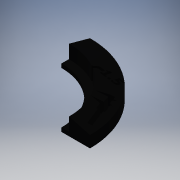
# Autodesk Inventor part: Mentor-CAD ring
Saved by Autodesk Inventor 2016 (Build 200138000, 138)
## iProperties
Created: 2016-02-20
Part Number: Mentor-CAD ring
Material: Generic
Document SubType Name: Modeling
Designer: RoksBot
Density: 1 g/cm^3
Appearance: Fine Textured - Black
Author: RoksBot
Autodesk Inventor part; units mm, degrees
ref_plane "YZ Plane" through (0, 0, 0) normal (1, 0, 0) x (0, 1, 0)
ref_plane "XZ Plane" through (0, 0, 0) normal (0, 1, 0) x (-1, 0, 0)
ref_plane "XY Plane" through (0, 0, 0) normal (0, 0, 1) x (1, 0, 0)
sketch "Sketch1" plane through (0, 0, 0) normal (0, 0, 1) x (1, 0, 0)
  line L0 (0, 0) -> (0, 8.6646) construction
  line L1 (20.9931, 1.27) -> (20.9931, 5.715)
  line L2 (20.9931, 5.715) -> (27.9781, 3.81)
  line L3 (27.9781, 3.81) -> (27.9781, 0)
  line L4 (27.9781, 0) -> (20.9931, 0)
  line L5 (20.9931, 1.27) -> (18.4531, 1.27)
  line L6 (18.4531, 1.27) -> (18.4531, 0)
  line L7 (18.4531, 0) -> (20.9931, 0)
  dimension "d0" = 20.9931
  dimension "d1" = 4.445
  dimension "d2" = 1.27
  dimension "d3" = 2.54
  dimension "d4" = 3.81
  dimension "d5" = 6.985
  constraints: 16 end point, 2 parallel, 2 perpendicular, 2 vertical, 1 horizontal, 1 horizontal alignment
  measures "d0" distance between parallel lines of L0 L1
  measures "d1" distance from line of L5 L1.end
  measures "d2" distance of L5.end L6.end
  measures "d3" distance between parallel lines of L1 L6
  measures "d4" distance of L2.end L3.end
  measures "d5" distance between parallel lines of L1 L3
revolve "Revolution1" add sketch "Sketch1" angle 360 about axis through (0, 0, 0) along (0, 1, 0)
sketch "Sketch2" plane through (0, 1.27, 0) normal (0, 1, 0) x (1, 0, 0)
  circle A0 centre (0, 0) radius 20.9931 projected
  circle A1 centre (0, 0) radius 27.9781 projected
  circle A2 centre (0, 0) radius 18.4531 projected
  line L0 (-4.2505, -7.1349) -> (4.1315, -7.1349) projected
  circle A3 centre (0, 0) radius 19.685 projected
  line L1 (-12.7595, -2.2222) -> (-12.7595, -29.7716) construction
  line L2 (12.6405, -2.2222) -> (12.6405, -30.8961) construction
  line L3 (-12.7549, -7.1349) -> (-31.6502, -7.1349) construction
  line L4 (0, 0) -> (17.3317, 30.0193) construction
  line L5 (-18.5741, 9.7833) -> (-25.4, 9.7833)
  line L6 (-18.8949, 9.1483) -> (-25.4, 9.1483)
  line L7 (-25.4, 9.1483) -> (-25.4, 9.7833)
  line L8 (-19.8553, -6.8174) -> (-25.4, -6.8174)
  line L9 (-25.4, -6.8174) -> (-25.4, -7.4524)
  line L10 (-25.4, -7.4524) -> (-19.6258, -7.4524)
  line L11 (0.1351, 9.4658) -> (-31.517, 9.4658) construction
  line L12 (-24.13, 9.1483) -> (-22.86, 6.9486)
  line L13 (-22.86, 6.9486) -> (-25.4, 6.9486)
  line L14 (-25.4, 6.9486) -> (-24.13, 9.1483)
  line L15 (-24.13, -6.8174) -> (-25.4, -4.6177)
  line L16 (-25.4, -4.6177) -> (-22.86, -4.6177)
  line L17 (-22.86, -4.6177) -> (-24.13, -6.8174)
  line L18 (-29.0818, 1.1654) -> (-16.5563, 1.1654) construction
  line L19 (-24.13, 7.6818) -> (-24.13, -5.3509) construction
  line L20 (-23.8125, 2.4354) -> (-24.4475, 2.4354)
  line L21 (-24.4475, 2.4354) -> (-24.4475, 6.9486)
  line L22 (-24.4475, 6.9486) -> (-23.8125, 6.9486)
  line L23 (-23.8125, 6.9486) -> (-23.8125, 2.4354)
  line L24 (-23.8125, 2.4354) -> (-24.4475, 6.9486) construction
  line L25 (-24.4475, 2.4354) -> (-23.8125, 6.9486) construction
  line L26 (-23.8125, -0.1046) -> (-24.4475, -0.1046)
  line L27 (-24.4475, -0.1046) -> (-24.4475, -4.6177)
  line L28 (-24.4475, -4.6177) -> (-23.8125, -4.6177)
  line L29 (-23.8125, -4.6177) -> (-23.8125, -0.1046)
  line L30 (-23.8125, -0.1046) -> (-24.4475, -4.6177) construction
  line L31 (-24.4475, -0.1046) -> (-23.8125, -4.6177) construction
  line L32 (-13.077, -16.4226) -> (-13.077, -23.7886)
  line L33 (-13.077, -23.7886) -> (-12.442, -23.7886)
  line L34 (-12.442, -23.7886) -> (-12.442, -16.9088)
  line L35 (12.323, -16.9957) -> (12.323, -23.7886)
  line L36 (12.323, -23.7886) -> (12.958, -23.7886)
  line L37 (12.958, -23.7886) -> (12.958, -16.5167)
  line L38 (-12.442, -22.5186) -> (-10.2423, -21.2486)
  line L39 (-10.2423, -21.2486) -> (-10.2423, -23.7886)
  line L40 (-10.2423, -23.7886) -> (-12.442, -22.5186)
  line L41 (12.323, -22.5186) -> (10.1233, -23.7886)
  line L42 (10.1233, -23.7886) -> (10.1233, -21.2486)
  line L43 (10.1233, -21.2486) -> (12.323, -22.5186)
  line L44 (-3.8695, -21.2486) -> (3.7505, -21.2486) construction
  line L45 (3.7505, -21.2486) -> (3.7505, -23.7886) construction
  line L46 (3.7505, -23.7886) -> (-3.8695, -23.7886) construction
  line L47 (-3.8695, -23.7886) -> (-3.8695, -21.2486) construction
  line L48 (-0.0595, -13.6296) -> (-0.0595, -32.797) construction
  line L49 (-10.2423, -22.5186) -> (10.1233, -22.5186) construction
  line L50 (-4.2505, -22.8361) -> (-10.2423, -22.8361)
  line L51 (-10.2423, -22.8361) -> (-10.2423, -22.2011)
  line L52 (-10.2423, -22.2011) -> (-4.2505, -22.2011)
  line L53 (-4.2505, -22.2011) -> (-4.2505, -22.8361)
  line L54 (-4.2505, -22.8361) -> (-10.2423, -22.2011) construction
  line L55 (-10.2423, -22.8361) -> (-4.2505, -22.2011) construction
  line L56 (4.1315, -22.2011) -> (10.1233, -22.2011)
  line L57 (10.1233, -22.2011) -> (10.1233, -22.8361)
  line L58 (10.1233, -22.8361) -> (4.1315, -22.8361)
  line L59 (4.1315, -22.8361) -> (4.1315, -22.2011)
  line L60 (4.1315, -22.2011) -> (10.1233, -22.8361) construction
  line L61 (10.1233, -22.2011) -> (4.1315, -22.8361) construction
  line L62 (10.1092, 18.3987) -> (11.0395, 20.0101)
  line L63 (11.0395, 20.0101) -> (11.8094, 19.5656)
  line L64 (11.8094, 19.5656) -> (10.8791, 17.9542)
  line L65 (12.9001, 20.8356) -> (18.6151, 20.8356) construction
  line L66 (18.6151, 20.8356) -> (18.6151, 18.2956) construction
  line L67 (18.6151, 18.2956) -> (12.9001, 18.2956) construction
  line L68 (12.9001, 18.2956) -> (12.9001, 20.8356) construction
  line L69 (11.0395, 20.0101) -> (12.9001, 20.0101)
  line L70 (12.9001, 20.0101) -> (12.9001, 19.1211)
  line L71 (12.9001, 19.1211) -> (11.0395, 19.1211)
  line L72 (11.0395, 19.1211) -> (11.0395, 20.0101)
  line L73 (11.0395, 20.0101) -> (12.9001, 19.1211) construction
  line L74 (12.9001, 20.0101) -> (11.0395, 19.1211) construction
  circle A4 centre (0, 0) radius 22.8981 construction
  line L75 (11.4654, -8.564) -> (6.3194, -8.564) projected
  line L76 (-26.9128, 0.2129) -> (-27.3651, 0.2129)
  line L77 (-27.3651, 0.2129) -> (-27.3651, 0.7162)
  line L78 (-27.3651, 0.7162) -> (-26.9128, 0.7162)
  line L79 (-26.9128, 0.7162) -> (-26.9128, 0.2129)
  spline S0 degree 2 poles (-25.1468, 0.8613) (-25.1468, 0.5603) (-25.5281, 0.1728) (-25.8615, 0.1728) knots 0 0 0 1 2 2 2
  spline S1 degree 2 poles (-25.8615, 0.1728) (-26.0282, 0.1728) (-26.2891, 0.2685) (-26.3802, 0.3627) knots 0 0 0 1 2 2 2
  spline S2 degree 2 poles (-26.3802, 0.3627) (-26.4883, 0.4723) (-26.6041, 0.8196) (-26.6041, 1.062) knots 0 0 0 1 2 2 2
  spline S3 degree 2 poles (-26.6041, 1.062) (-26.6041, 1.3121) (-26.496, 1.7011) (-26.374, 1.8509) knots 0 0 0 1 2 2 2
  spline S4 degree 2 poles (-26.374, 1.8509) (-26.2583, 1.9929) (-25.8816, 2.1535) (-25.6238, 2.1535) knots 0 0 0 1 2 2 2
  spline S5 degree 2 poles (-25.6238, 2.1535) (-25.5296, 2.1535) (-25.3413, 2.1288) (-25.3073, 2.121) knots 0 0 0 1 2 2 2
  line L80 (-25.3073, 2.121) -> (-25.3073, 1.7474)
  line L81 (-25.3073, 1.7474) -> (-25.3413, 1.7474)
  spline S6 degree 2 poles (-25.3413, 1.7474) (-25.3752, 1.7644) (-25.5296, 1.8061) (-25.6284, 1.8061) knots 0 0 0 1 2 2 2
  spline S7 degree 2 poles (-25.6284, 1.8061) (-25.8523, 1.8061) (-26.0962, 1.5699) (-26.1255, 1.3507) knots 0 0 0 1 2 2 2
  spline S8 degree 2 poles (-26.1255, 1.3507) (-26.0313, 1.4109) (-25.8384, 1.4819) (-25.7164, 1.4819) knots 0 0 0 1 2 2 2
  spline S9 degree 2 poles (-25.7164, 1.4819) (-25.613, 1.4819) (-25.4324, 1.4263) (-25.3629, 1.3739) knots 0 0 0 1 2 2 2
  spline S10 degree 2 poles (-25.3629, 1.3739) (-25.2641, 1.2982) (-25.1468, 1.0528) (-25.1468, 0.8613) knots 0 0 0 1 2 2 2
  spline S11 degree 2 poles (-25.7041, 0.5742) (-25.667, 0.6205) (-25.6269, 0.7286) (-25.6269, 0.8382) knots 0 0 0 1 2 2 2
  spline S12 degree 2 poles (-25.6269, 0.8382) (-25.6269, 0.9308) (-25.6732, 1.0512) (-25.7149, 1.0867) knots 0 0 0 1 2 2 2
  spline S13 degree 2 poles (-25.7149, 1.0867) (-25.7581, 1.1238) (-25.8646, 1.15) (-25.9248, 1.15) knots 0 0 0 1 2 2 2
  spline S14 degree 2 poles (-25.9248, 1.15) (-25.9758, 1.15) (-26.0807, 1.1238) (-26.127, 1.1052) knots 0 0 0 1 2 2 2
  spline S15 degree 2 poles (-26.127, 1.1052) (-26.127, 1.0929) (-26.1301, 1.0342) (-26.1301, 0.9895) knots 0 0 0 1 2 2 2
  spline S16 degree 2 poles (-26.1301, 0.9895) (-26.1301, 0.8243) (-26.073, 0.6251) (-26.0282, 0.5742) knots 0 0 0 1 2 2 2
  spline S17 degree 2 poles (-26.0282, 0.5742) (-25.9958, 0.5325) (-25.9094, 0.497) (-25.8631, 0.497) knots 0 0 0 1 2 2 2
  spline S18 degree 2 poles (-25.8631, 0.497) (-25.8245, 0.497) (-25.7349, 0.5356) (-25.7041, 0.5742) knots 0 0 0 1 2 2 2
  spline S19 degree 2 poles (-23.5104, 0.8582) (-23.5104, 0.7085) (-23.6123, 0.4553) (-23.7126, 0.3642) knots 0 0 0 1 2 2 2
  spline S20 degree 2 poles (-23.7126, 0.3642) (-23.8129, 0.2732) (-24.0877, 0.1728) (-24.2884, 0.1728) knots 0 0 0 1 2 2 2
  spline S21 degree 2 poles (-24.2884, 0.1728) (-24.5015, 0.1744) (-24.8071, 0.2438) (-24.9075, 0.2886) knots 0 0 0 1 2 2 2
  line L82 (-24.9075, 0.2886) -> (-24.9075, 0.7039)
  line L83 (-24.9075, 0.7039) -> (-24.8643, 0.7039)
  spline S22 degree 2 poles (-24.8643, 0.7039) (-24.8272, 0.6838) (-24.7377, 0.6313) (-24.6651, 0.6035) knots 0 0 0 1 2 2 2
  spline S23 degree 2 poles (-24.6651, 0.6035) (-24.5972, 0.5773) (-24.4567, 0.5418) (-24.3718, 0.5418) knots 0 0 0 1 2 2 2
  spline S24 degree 2 poles (-24.3718, 0.5418) (-24.2977, 0.5418) (-24.1248, 0.5788) (-24.0723, 0.6282) knots 0 0 0 1 2 2 2
  spline S25 degree 2 poles (-24.0723, 0.6282) (-24.0337, 0.6668) (-23.9905, 0.761) (-23.9905, 0.8397) knots 0 0 0 1 2 2 2
  spline S26 degree 2 poles (-23.9905, 0.8397) (-23.9905, 0.9076) (-24.0461, 1.0034) (-24.0908, 1.0327) knots 0 0 0 1 2 2 2
  spline S27 degree 2 poles (-24.0908, 1.0327) (-24.1557, 1.0759) (-24.3409, 1.1006) (-24.4073, 1.1006) knots 0 0 0 1 2 2 2
  spline S28 degree 2 poles (-24.4073, 1.1006) (-24.5123, 1.1006) (-24.7114, 1.0666) (-24.784, 1.0481) knots 0 0 0 1 2 2 2
  line L84 (-24.784, 1.0481) -> (-24.8257, 1.0481)
  line L85 (-24.8257, 1.0481) -> (-24.8257, 2.1179)
  line L86 (-24.8257, 2.1179) -> (-23.5629, 2.1179)
  line L87 (-23.5629, 2.1179) -> (-23.5629, 1.7583)
  line L88 (-23.5629, 1.7583) -> (-24.3733, 1.7583)
  line L89 (-24.3733, 1.7583) -> (-24.3733, 1.4418)
  spline S29 degree 2 poles (-24.3733, 1.4418) (-24.3347, 1.4449) (-24.2282, 1.448) (-24.1989, 1.448) knots 0 0 0 1 2 2 2
  spline S30 degree 2 poles (-24.1989, 1.448) (-24.0615, 1.448) (-23.8299, 1.3924) (-23.7388, 1.3353) knots 0 0 0 1 2 2 2
  spline S31 degree 2 poles (-23.7388, 1.3353) (-23.6308, 1.2642) (-23.5104, 1.0281) (-23.5104, 0.8582) knots 0 0 0 1 2 2 2
  line L90 (-21.7752, 0.6575) -> (-22.033, 0.6575)
  line L91 (-22.033, 0.6575) -> (-22.033, 0.2083)
  line L92 (-22.033, 0.2083) -> (-22.4946, 0.2083)
  line L93 (-22.4946, 0.2083) -> (-22.4946, 0.6575)
  line L94 (-22.4946, 0.6575) -> (-23.3344, 0.6575)
  line L95 (-23.3344, 0.6575) -> (-23.3344, 1.0126)
  line L96 (-23.3344, 1.0126) -> (-22.51, 2.1179)
  line L97 (-22.51, 2.1179) -> (-22.033, 2.1179)
  line L98 (-22.033, 2.1179) -> (-22.033, 1.0003)
  line L99 (-22.033, 1.0003) -> (-21.7752, 1.0003)
  line L100 (-21.7752, 1.0003) -> (-21.7752, 0.6575)
  line L101 (-22.4946, 1.0003) -> (-22.4946, 1.6486)
  line L102 (-22.4946, 1.6486) -> (-22.9778, 1.0003)
  line L103 (-22.9778, 1.0003) -> (-22.4946, 1.0003)
  line L104 (-2.2979, -23.4704) -> (-3.5561, -23.4704)
  line L105 (-3.5561, -23.4704) -> (-3.5561, -23.1385)
  line L106 (-3.5561, -23.1385) -> (-3.1547, -23.1385)
  line L107 (-3.1547, -23.1385) -> (-3.1547, -22.1304)
  line L108 (-3.1547, -22.1304) -> (-3.5561, -22.1304)
  line L109 (-3.5561, -22.1304) -> (-3.5561, -21.8201)
  spline S32 degree 2 poles (-3.5561, -21.8201) (-3.4681, -21.8201) (-3.2937, -21.7969) (-3.2412, -21.7722) knots 0 0 0 1 2 2 2
  spline S33 degree 2 poles (-3.2412, -21.7722) (-3.181, -21.7413) (-3.113, -21.6379) (-3.1069, -21.5607) knots 0 0 0 1 2 2 2
  line L110 (-3.1069, -21.5607) -> (-2.69, -21.5607)
  line L111 (-2.69, -21.5607) -> (-2.69, -23.1385)
  line L112 (-2.69, -23.1385) -> (-2.2979, -23.1385)
  line L113 (-2.2979, -23.1385) -> (-2.2979, -23.4704)
  line L114 (-1.5029, -23.4704) -> (-1.9552, -23.4704)
  line L115 (-1.9552, -23.4704) -> (-1.9552, -22.9671)
  line L116 (-1.9552, -22.9671) -> (-1.5029, -22.9671)
  line L117 (-1.5029, -22.9671) -> (-1.5029, -23.4704)
  spline S34 degree 2 poles (0.2493, -22.5179) (0.2493, -22.7649) (0.1705, -23.1354) (0.0825, -23.2604) knots 0 0 0 1 2 2 2
  spline S35 degree 2 poles (0.0825, -23.2604) (-0.0039, -23.3839) (-0.2833, -23.5105) (-0.484, -23.5105) knots 0 0 0 1 2 2 2
  spline S36 degree 2 poles (-0.484, -23.5105) (-0.6862, -23.5105) (-0.9641, -23.3839) (-1.0521, -23.2573) knots 0 0 0 1 2 2 2
  spline S37 degree 2 poles (-1.0521, -23.2573) (-1.1401, -23.1323) (-1.2188, -22.7649) (-1.2188, -22.5179) knots 0 0 0 1 2 2 2
  spline S38 degree 2 poles (-1.2188, -22.5179) (-1.2188, -22.2647) (-1.1401, -21.9065) (-1.0506, -21.7769) knots 0 0 0 1 2 2 2
  spline S39 degree 2 poles (-1.0506, -21.7769) (-0.961, -21.6503) (-0.6785, -21.5268) (-0.484, -21.5268) knots 0 0 0 1 2 2 2
  spline S40 degree 2 poles (-0.484, -21.5268) (-0.2787, -21.5268) (-0.0039, -21.6564) (0.0841, -21.7846) knots 0 0 0 1 2 2 2
  spline S41 degree 2 poles (0.0841, -21.7846) (0.1705, -21.9096) (0.2493, -22.2786) (0.2493, -22.5179) knots 0 0 0 1 2 2 2
  spline S42 degree 2 poles (-0.2308, -22.5179) (-0.2308, -22.1643) (-0.3466, -21.8787) (-0.484, -21.8787) knots 0 0 0 1 2 2 2
  spline S43 degree 2 poles (-0.484, -21.8787) (-0.6214, -21.8787) (-0.7387, -22.1643) (-0.7387, -22.5194) knots 0 0 0 1 2 2 2
  spline S44 degree 2 poles (-0.7387, -22.5194) (-0.7387, -22.8683) (-0.6214, -23.1585) (-0.484, -23.1585) knots 0 0 0 1 2 2 2
  spline S45 degree 2 poles (-0.484, -23.1585) (-0.3482, -23.1585) (-0.2308, -22.8683) (-0.2308, -22.5179) knots 0 0 0 1 2 2 2
  spline S46 degree 2 poles (1.9181, -22.5179) (1.9181, -22.7649) (1.8393, -23.1354) (1.7513, -23.2604) knots 0 0 0 1 2 2 2
  spline S47 degree 2 poles (1.7513, -23.2604) (1.6649, -23.3839) (1.3855, -23.5105) (1.1848, -23.5105) knots 0 0 0 1 2 2 2
  spline S48 degree 2 poles (1.1848, -23.5105) (0.9826, -23.5105) (0.7047, -23.3839) (0.6167, -23.2573) knots 0 0 0 1 2 2 2
  spline S49 degree 2 poles (0.6167, -23.2573) (0.5287, -23.1323) (0.45, -22.7649) (0.45, -22.5179) knots 0 0 0 1 2 2 2
  spline S50 degree 2 poles (0.45, -22.5179) (0.45, -22.2647) (0.5287, -21.9065) (0.6182, -21.7769) knots 0 0 0 1 2 2 2
  spline S51 degree 2 poles (0.6182, -21.7769) (0.7078, -21.6503) (0.9903, -21.5268) (1.1848, -21.5268) knots 0 0 0 1 2 2 2
  spline S52 degree 2 poles (1.1848, -21.5268) (1.3901, -21.5268) (1.6649, -21.6564) (1.7529, -21.7846) knots 0 0 0 1 2 2 2
  spline S53 degree 2 poles (1.7529, -21.7846) (1.8393, -21.9096) (1.9181, -22.2786) (1.9181, -22.5179) knots 0 0 0 1 2 2 2
  spline S54 degree 2 poles (1.438, -22.5179) (1.438, -22.1643) (1.3222, -21.8787) (1.1848, -21.8787) knots 0 0 0 1 2 2 2
  spline S55 degree 2 poles (1.1848, -21.8787) (1.0474, -21.8787) (0.9301, -22.1643) (0.9301, -22.5194) knots 0 0 0 1 2 2 2
  spline S56 degree 2 poles (0.9301, -22.5194) (0.9301, -22.8683) (1.0474, -23.1585) (1.1848, -23.1585) knots 0 0 0 1 2 2 2
  spline S57 degree 2 poles (1.1848, -23.1585) (1.3206, -23.1585) (1.438, -22.8683) (1.438, -22.5179) knots 0 0 0 1 2 2 2
  spline S58 degree 2 poles (3.5869, -22.5179) (3.5869, -22.7649) (3.5081, -23.1354) (3.4202, -23.2604) knots 0 0 0 1 2 2 2
  spline S59 degree 2 poles (3.4202, -23.2604) (3.3337, -23.3839) (3.0543, -23.5105) (2.8536, -23.5105) knots 0 0 0 1 2 2 2
  spline S60 degree 2 poles (2.8536, -23.5105) (2.6514, -23.5105) (2.3735, -23.3839) (2.2855, -23.2573) knots 0 0 0 1 2 2 2
  spline S61 degree 2 poles (2.2855, -23.2573) (2.1975, -23.1323) (2.1188, -22.7649) (2.1188, -22.5179) knots 0 0 0 1 2 2 2
  spline S62 degree 2 poles (2.1188, -22.5179) (2.1188, -22.2647) (2.1975, -21.9065) (2.287, -21.7769) knots 0 0 0 1 2 2 2
  spline S63 degree 2 poles (2.287, -21.7769) (2.3766, -21.6503) (2.6591, -21.5268) (2.8536, -21.5268) knots 0 0 0 1 2 2 2
  spline S64 degree 2 poles (2.8536, -21.5268) (3.0589, -21.5268) (3.3337, -21.6564) (3.4217, -21.7846) knots 0 0 0 1 2 2 2
  spline S65 degree 2 poles (3.4217, -21.7846) (3.5081, -21.9096) (3.5869, -22.2786) (3.5869, -22.5179) knots 0 0 0 1 2 2 2
  spline S66 degree 2 poles (3.1068, -22.5179) (3.1068, -22.1643) (2.991, -21.8787) (2.8536, -21.8787) knots 0 0 0 1 2 2 2
  spline S67 degree 2 poles (2.8536, -21.8787) (2.7162, -21.8787) (2.5989, -22.1643) (2.5989, -22.5194) knots 0 0 0 1 2 2 2
  spline S68 degree 2 poles (2.5989, -22.5194) (2.5989, -22.8683) (2.7162, -23.1585) (2.8536, -23.1585) knots 0 0 0 1 2 2 2
  spline S69 degree 2 poles (2.8536, -23.1585) (2.9894, -23.1585) (3.1068, -22.8683) (3.1068, -22.5179) knots 0 0 0 1 2 2 2
  line L118 (14.9222, 18.1946) -> (13.0768, 18.1946)
  line L119 (13.0768, 18.1946) -> (13.0768, 18.6814)
  line L120 (13.0768, 18.6814) -> (13.6655, 18.6814)
  line L121 (13.6655, 18.6814) -> (13.6655, 20.1599)
  line L122 (13.6655, 20.1599) -> (13.0768, 20.1599)
  line L123 (13.0768, 20.1599) -> (13.0768, 20.615)
  spline S70 degree 2 poles (13.0768, 20.615) (13.2059, 20.615) (13.4618, 20.649) (13.5387, 20.6852) knots 0 0 0 1 2 2 2
  spline S71 degree 2 poles (13.5387, 20.6852) (13.627, 20.7305) (13.7267, 20.8822) (13.7357, 20.9954) knots 0 0 0 1 2 2 2
  line L124 (13.7357, 20.9954) -> (14.3471, 20.9954)
  line L125 (14.3471, 20.9954) -> (14.3471, 18.6814)
  line L126 (14.3471, 18.6814) -> (14.9222, 18.6814)
  line L127 (14.9222, 18.6814) -> (14.9222, 18.1946)
  line L128 (16.0882, 18.1946) -> (15.4248, 18.1946)
  line L129 (15.4248, 18.1946) -> (15.4248, 18.9327)
  line L130 (15.4248, 18.9327) -> (16.0882, 18.9327)
  line L131 (16.0882, 18.9327) -> (16.0882, 18.1946)
  spline S72 degree 2 poles (18.6309, 19.141) (18.6309, 18.9214) (18.4814, 18.5501) (18.3343, 18.4165) knots 0 0 0 1 2 2 2
  spline S73 degree 2 poles (18.3343, 18.4165) (18.1871, 18.2829) (17.7841, 18.1357) (17.4897, 18.1357) knots 0 0 0 1 2 2 2
  spline S74 degree 2 poles (17.4897, 18.1357) (17.1773, 18.138) (16.729, 18.2399) (16.5818, 18.3055) knots 0 0 0 1 2 2 2
  line L132 (16.5818, 18.3055) -> (16.5818, 18.9146)
  line L133 (16.5818, 18.9146) -> (16.6452, 18.9146)
  spline S75 degree 2 poles (16.6452, 18.9146) (16.6995, 18.8852) (16.8309, 18.8082) (16.9373, 18.7674) knots 0 0 0 1 2 2 2
  spline S76 degree 2 poles (16.9373, 18.7674) (17.0369, 18.7289) (17.2429, 18.6769) (17.3675, 18.6769) knots 0 0 0 1 2 2 2
  spline S77 degree 2 poles (17.3675, 18.6769) (17.4762, 18.6769) (17.7297, 18.7312) (17.8067, 18.8037) knots 0 0 0 1 2 2 2
  spline S78 degree 2 poles (17.8067, 18.8037) (17.8633, 18.8603) (17.9267, 18.9984) (17.9267, 19.1138) knots 0 0 0 1 2 2 2
  spline S79 degree 2 poles (17.9267, 19.1138) (17.9267, 19.2135) (17.8452, 19.3539) (17.7796, 19.3969) knots 0 0 0 1 2 2 2
  spline S80 degree 2 poles (17.7796, 19.3969) (17.6845, 19.4603) (17.4128, 19.4965) (17.3154, 19.4965) knots 0 0 0 1 2 2 2
  spline S81 degree 2 poles (17.3154, 19.4965) (17.1614, 19.4965) (16.8694, 19.4467) (16.7629, 19.4195) knots 0 0 0 1 2 2 2
  line L134 (16.7629, 19.4195) -> (16.7018, 19.4195)
  line L135 (16.7018, 19.4195) -> (16.7018, 20.9886)
  line L136 (16.7018, 20.9886) -> (18.5539, 20.9886)
  line L137 (18.5539, 20.9886) -> (18.5539, 20.461)
  line L138 (18.5539, 20.461) -> (17.3652, 20.461)
  line L139 (17.3652, 20.461) -> (17.3652, 19.9969)
  spline S82 degree 2 poles (17.3652, 19.9969) (17.4218, 20.0014) (17.578, 20.0059) (17.6211, 20.0059) knots 0 0 0 1 2 2 2
  spline S83 degree 2 poles (17.6211, 20.0059) (17.8226, 20.0059) (18.1622, 19.9244) (18.2958, 19.8407) knots 0 0 0 1 2 2 2
  spline S84 degree 2 poles (18.2958, 19.8407) (18.4543, 19.7365) (18.6309, 19.3901) (18.6309, 19.141) knots 0 0 0 1 2 2 2
  point P0 (-10.4828, 14.7667)
  point P1 (-24.13, 4.692)
  point P2 (-24.13, -2.3611)
  point P3 (-10.9755, -22.5186)
  point P4 (10.8565, -22.5186)
  point P5 (-3.8695, -22.5186)
  point P6 (-0.0595, -23.7886)
  point P7 (-7.2464, -22.5186)
  point P8 (7.1274, -22.5186)
  point P9 (11.9698, 19.5656)
  point P10 (11.9698, 19.5656)
  point P11 (18.6151, 19.5656)
  dimension "d7" = 39.37
  dimension "d9" = 25.4
  dimension "d11" = 0.635
  dimension "d13" = 25.4
  dimension "d14" = 0.635
  dimension "d15" = 0.3175
  dimension "d16" = 16.6007
  dimension "d17" = 0.3175
  dimension "d18" = 2.54
  dimension "d19" = 1.27
  dimension "d20" = 1.27
  dimension "d21" = 0.635
  dimension "d22" = 0.3175
  dimension "d23" = 7.366
  dimension "d24" = 0.3175
  dimension "d25" = 2.54
  dimension "d26" = 7.62
  dimension "d27" = 2.54
  dimension "d28" = 0.635
  dimension "d29" = 0.381
  dimension "d30" = 0.381
  dimension "d31" = 0.889
  dimension "d32" = 0.4445
  dimension "d33" = 5.715
  dimension "d34" = 2.54
  dimension "d35" = 27.94
  dimension "d36" = 0.889
  dimension "d38" = 60
  dimension "d39" = 1.905
  constraints: 132 end point, 16 midpoint, 16 point on line, 14 perpendicular, 13 horizontal, 12 parallel, 8 vertical, 5 equal length, 5 horizontal alignment, 3 vertical alignment, 1 centre point, 1 coincident, 1 collinear, 49 other
  measures "d7" diameter of A3
  measures "d9" distance between parallel lines of L2 L1
  measures "d11" distance between parallel lines of L6 L5
  measures "d13" horizontal distance of A1.centre L5.end
  measures "d14" distance between parallel lines of L10 L8
  measures "d15" distance between parallel lines of L10 L3
  measures "d16" distance from line of L11.start L0
  measures "d17" distance between parallel lines of L11 L5
  measures "d18" distance of L12.end L13.end
  measures "d19" distance between parallel lines of L18 L20
  measures "d20" distance between parallel lines of L18 L26
  measures "d21" distance of L32.end L33.end
  measures "d22" distance between parallel lines of L1 L32
  measures "d23" distance of L32.start L32.end
  measures "d24" distance between parallel lines of L2 L35
  measures "d25" distance of L38.end L39.end
  measures "d26" distance of L45.end L46.end
  measures "d27" distance of L44.end L45.end
  measures "d28" distance of L52.end L50.start
  measures "d29" distance between parallel lines of L47 L53
  measures "d30" distance between parallel lines of L45 L59
  measures "d31" distance of L62.end L63.end
  measures "d32" distance between parallel lines of L4 L62
  measures "d33" distance of L65.start L65.end
  measures "d34" distance of L65.end L66.end
  measures "d35" distance of A1.centre L65.end
  measures "d36" distance of L69.end L70.end
  measures "d38" angle of L0 L4
extrude "Extrusion1" cut sketch "Sketch2" along normal through all contours L41 L42 L43 | L38 L39 L40 | L15 L16 L17 | L12 L13 L14 | A0 L62 L72 L71 L64 | L37 L36 L35 A0 | L71 L72 L63 L64 | L64 L63 L69 L70 L71 | A0 L6 L7 L5 | L34 L33 L32 A0 | A0 L10 L9 L8 | L58 L59 L56 L42 | L52 L53 L50 L39 | L23 L20 L21 L13 | L27 L26 L29 L16 | L137 L138 L139 S82 S83 S84 S72 S73 S74 L132 L133 S75 S76 S77 S78 S79 S80 S81 L134 L135 L136 A1 | A1 L136 L137 | L76 L77 L78 L79 | S0 S1 S2 S3 S4 S5 L80 L81 S6 S7 S8 S9 S10 | S19 S20 S21 L82 L83 S22 S23 S24 S25 S26 S27 S28 L84 L85 L86 L87 L88 L89 S29 S30 S31 | L90 L91 L92 L93 L94 L95 L96 L97 L98 L99 L100 | L104 L105 L106 L107 L108 L109 S32 S33 L110 L111 L112 L113 | L114 L115 L116 L117 | S34 S35 S36 S37 S38 S39 S40 S41 | S46 S47 S48 S49 S50 S51 S52 S53 | S58 S59 S60 S61 S62 S63 S64 S65 | L118 L119 L120 L121 L122 L123 S70 S71 L124 L125 L126 L127 | L128 L129 L130 L131 picked at (16.9229, 20.135)
sketch "Sketch3" plane through (-25.4, 1.27, -9.7833) normal (0, 1, 0) x (1, 0, 0)
  circle A0 centre (25.4, -9.7833) radius 18.415 projected
  circle A1 centre (25.4, -9.7833) radius 19.685 projected
  circle A2 centre (25.4, -9.7833) radius 27.9781 projected
  line L0 (51.4124, -7.0731) -> (47.0687, 4.861)
  line L1 (47.0687, 4.861) -> (45.8753, 4.4266)
  line L2 (45.8753, 4.4266) -> (50.219, -7.5075)
  line L3 (50.219, -7.5075) -> (51.4124, -7.0731)
  line L4 (51.4124, -7.0731) -> (45.8753, 4.4266) construction
  line L5 (47.0687, 4.861) -> (50.219, -7.5075) construction
  line L6 (46.6739, 0.933) -> (47.7598, -2.0505)
  line L7 (47.7598, -2.0505) -> (49.7886, -1.3121)
  line L8 (49.7886, -1.3121) -> (48.7026, 1.6715)
  line L9 (48.7026, 1.6715) -> (46.6739, 0.933)
  line L10 (46.6739, 0.933) -> (49.7886, -1.3121) construction
  line L11 (47.7598, -2.0505) -> (48.7026, 1.6715) construction
  line L12 (45.8753, 4.4266) -> (43.2393, 2.386)
  line L13 (43.2393, 2.386) -> (46.2228, 3.4719)
  line L14 (46.6739, 0.933) -> (44.108, -0.0008)
  line L15 (44.108, -0.0008) -> (47.0213, -0.0217)
  line L16 (47.4162, 3.9063) -> (48.371, 4.2538)
  line L17 (48.371, 4.2538) -> (47.6334, 3.3096)
  line L18 (25.4, -9.7833) -> (37.7185, -9.7833) construction
  line L19 (48.7026, 1.6715) -> (49.2397, 1.8669)
  line L20 (49.2397, 1.8669) -> (48.0678, 2.1161)
  line L21 (48.0678, 2.1161) -> (48.285, 1.5194) construction
  point P0 (48.6439, -1.3232)
  point P1 (48.2312, -0.1895)
  dimension "d42" = 3.175
  dimension "d43" = 3.175
  dimension "d44" = 1.016
  dimension "d45" = 1.27
  dimension "d46" = 1.016
  dimension "d47" = 1.016
  dimension "d49" = 0.635
  dimension "d50" = 3.175
  dimension "d51" = 12.7
  dimension "d52" = 2.159
  dimension "d53" = 2.54
  dimension "d54" = 24.765
  dimension "d55" = 0.635
  dimension "d56" = 24.9231
  dimension "d57" = 24.9231
  dimension "d58" = 340
  dimension "d59" = 1.016
  dimension "d60" = 0.635
  constraints: 44 end point, 10 point on line, 6 parallel, 4 midpoint, 3 perpendicular, 1 horizontal
  measures "d42" distance from line of L2 L12.end
  measures "d43" distance from line of L2 L14.end
  measures "d44" distance of L6.start L15.end
  measures "d45" distance between parallel lines of L0 L2
  measures "d46" distance of L1.end L13.end
  measures "d47" distance of L16.start L16.end
  measures "d49" distance of L16.start L17.end
  measures "d50" distance of L7.end L8.end
  measures "d51" distance between parallel lines of L3 L1
  measures "d52" distance between parallel lines of L8 L6
  measures "d53" distance between parallel lines of L14 L13
  measures "d54" distance of point (25.4, -9.783) point (48.231, -0.19)
  measures "d55" distance from line of L0 point (48.231, -0.19)
  measures "d56" distance of A0.centre L1.end
  measures "d57" distance of A0.centre L2.end
  measures "d59" distance from line of L0 L19.end
  measures "d60" distance from line of L9 L20.end
extrude "Extrusion2" cut sketch "Sketch3" along normal through all contours L0 L9 L2 L1 | L20 L19 L9 L0 | L0 L16 L17 | L9 L8 L7 L0 | L0 L7 L2 L9 | L0 L3 L2 L7 | L2 L7 L6 L9 | L13 L12 L2 | L6 L15 L14
sketch "Sketch4" plane through (-25.4, 1.27, -9.7833) normal (0, 1, 0) x (1, 0, 0)
  line L0 (25.4, -9.7833) -> (64.551, -9.7833)
  line L1 (64.551, -9.7833) -> (64.551, 27.8106)
  line L2 (64.551, 27.8106) -> (25.4, 27.8106)
  line L3 (25.4, 27.8106) -> (25.4, -9.7833)
  constraints: 8 end point, 2 parallel, 1 horizontal, 1 perpendicular
extrude "Extrusion3" cut sketch "Sketch4" along normal through all both and the other way through all keep common part
equation "\"d15\" = 0.5 * d14"
equation "\"d17\" = 0.5 * d11"
equation "\"d22\" = 0.5 * d21"
equation "\"d24\" = d22"
equation "\"d32\" = 0.5 * d31"
body "Solid1"
